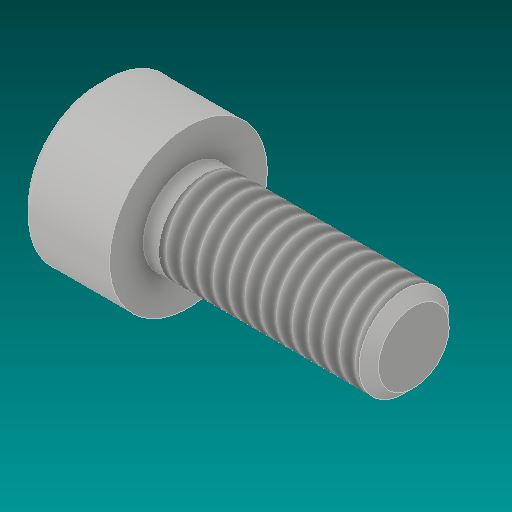
# Autodesk Inventor part: BOLT4-10
Saved by Autodesk Inventor 2020 (Build 240168000, 168)
## iProperties
Created: 2022-11-04
Part Number: BOLT4-10
Material: Generic
Catalog Web Link: www.cadenas.de
Description: BOLT-Hexagon Socket Head Cap Screws
Vendor: MISUMI
Document SubType Name: Modeling
Designer: psAdmin
Manufacturer: MISUMI
Mass: 0.260298 g
Surface Area: 3.02869 cm^2
Volume: 0.260298 cm^3
Density: 1 g/cm^3
Appearance: PSOLRGB-175-175-175
Category: PARTsolutions
Company: MISUMI
PSOL_IDENT_0: {$CADENAS_DATA/23d-libs/misumi/metric/accessories/bolt.prj},156 {VTYP=3D},{NB=BOLT4-10},{LINA=BOLT4-
PSOL_IDENT_1: 10},{NN=BOLT},{DATE=30.06.2021 13:30:08},{GEOMDATE=12.05.2017 08:21:09},{VERSION=},{LINEID=50},{WBVA
PSOL_IDENT_2: R=L},{WBNUMERIC=L}  {NB=BOLT4-10},{LINA=BOLT4-10},{KT=DUMMY},{PN=BOLT4-10},{TYPE=BOLT},{L=10.0},{M=4
PSOL_IDENT_3: .0},{P=0.7},{A=7.0},{E=4.0},{B=3.0},{C=0.40},{LL=0}
NB: BOLT4-10
NN: BOLT
NT: Hexagon Socket Head Cap Screws
NBSYN: $PN.
LINA: BOLT4-10
CATALOG: Misumi
PN: BOLT4-10
L: 10
M: 4
P: 0.7
C: 0.4
SUPPLIER: MISUMI
ARTICLENO: BOLT4-10
BOMINFO: BOLT4-10
CREATOR: CADENAS GmbH
d12: 0.000 mm
Title: BOLT4-10
Author: Cadenas PARTsolutions
Comments: Hexagon Socket Head Cap Screws
Autodesk Inventor part; units mm, degrees
sketch "Sketch_1" plane through (0, 0, 0) normal (0, 0, 1) x (1, 0, 0)
  line L0 (10, 0) -> (-4, 0)
  line L1 (-4, 0) -> (-4, 3.1)
  line L2 (-4, 3.1) -> (-3.6, 3.5)
  line L3 (-3.6, 3.5) -> (0, 3.5)
  line L4 (0, 3.5) -> (0, 2)
  line L5 (0, 2) -> (9.5705, 2)
  line L6 (9.5705, 2) -> (10, 1.5705)
  line L7 (10, 1.5705) -> (10, 0)
  line L8 (10, 0) -> (-4, 0)
  constraints: 18 end point
revolve "Revolution1" add sketch "Sketch_1" angle 360 about axis through (10, 0, 0) along (1, 0, 0)
thread "Thread1" size "M4x0.7" class "6g" standard "ISO Metric profile" length 8.8705
sketch "Sketch2" plane through (-4, 0, 0) normal (-1, 0, 0) x (0, 0, 1)
  point P0 (0, 0)
hole "Hole1" at (-4, 0, 0) direction (1, 0, 0) diameter 3 depth 2 tip angle 150
sketch "Sketch_3" plane through (-4, 0, 0) normal (1, 0, 0) x (0, 0, -1)
  line L0 (-1.5, -0.866) -> (0, -1.7321)
  line L1 (0, -1.7321) -> (1.5, -0.866)
  line L2 (1.5, -0.866) -> (1.5, 0.866)
  line L3 (1.5, 0.866) -> (0, 1.7321)
  line L4 (0, 1.7321) -> (-1.5, 0.866)
  line L5 (-1.5, 0.866) -> (-1.5, -0.866)
  constraints: 12 end point
extrude "Extrusion1" cut sketch "Sketch_3" along normal blind 2
ref_plane "to_cp_XY" through (0, 0, 0) normal (1, 0, 0) x (0, 0, -1)
ref_plane "to_cp_YZ" through (0, 0, 0) normal (0, 0, -1) x (0, 1, 0)
ref_plane "to_cp_ZX" through (0, 0, 0) normal (0, 1, 0) x (1, 0, 0)
body "Solid1"
